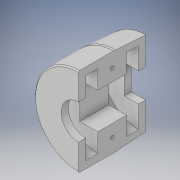
# Autodesk Inventor part: cameraHolder
Saved by Autodesk Inventor 2019.3 (Build 233278000, 278)
## iProperties
Created: 2019-10-29
Part Number: cameraHolder
Material: Generic
Document SubType Name: Modeling
Designer: Ayaz
Density: 1 g/cm^3
Appearance: Default
Author: Ayaz
Autodesk Inventor part; units mm, degrees
ref_plane "YZ Plane" through (0, 0, 0) normal (1, 0, 0) x (0, 1, 0)
ref_plane "XZ Plane" through (0, 0, 0) normal (0, 1, 0) x (-1, 0, 0)
ref_plane "XY Plane" through (0, 0, 0) normal (0, 0, 1) x (1, 0, 0)
sketch "Sketch1" plane through (0, 0, 0) normal (0, 1, 0) x (-1, 0, 0)
  line L0 (0, 0) -> (0, 36.83)
  line L1 (0, 0) -> (-56, 0)
  line L2 (-56, 0) -> (-56, 34.9885)
  line L3 (11.2, 0) -> (-67.2, 0) projected
  line L4 (-50, 30.1718) -> (-50, 6)
  line L5 (-6, 6) -> (-6, 30.7506)
  line L6 (-6, 30.7506) -> (-50, 30.1718)
  line L7 (-28, 0) -> (-28, 30.4612)
  line L8 (-16, 0) -> (-16, 30.619)
  line L9 (-40, 0) -> (-40, 30.3033)
  line L10 (-50, 6) -> (-40, 6)
  line L11 (-16, 6) -> (-6, 6)
  line L12 (0, 36.83) -> (-30, 36.83)
  line L13 (-30, 36.83) -> (-56, 34.9885)
  dimension "d1" = 34.9885
  dimension "d8" = 36.83
  dimension "d10" = 56
  dimension "d22" = 28
  dimension "d23" = 12
  dimension "d24" = 12
  dimension "d29" = 30
  constraints: 26 end point, 4 point on line, 2 midpoint, 2 parallel, 2 vertical, 1 horizontal, 1 perpendicular
  measures "d1" distance of L1.end L2.end
  measures "d8" distance of L0.start L0.end
  measures "d10" distance of L0.start L1.end
  measures "d22" distance between parallel lines of L0 L7
  measures "d23" distance between parallel lines of L7 L8
  measures "d24" distance between parallel lines of L7 L9
  measures "d29" distance of L0.end L12.end
revolve "Revolution1" add sketch "Sketch1" angle 180 about axis through (-10, 0, 0) along (-1, 0, 0) contours L1 L8 L11 L5 L6 L4 L10 L9 L2 L13 L12 L0 | L1 L7 L6 L8 | L1 L9 L6 L7
ref_plane "Work Plane1" through (6, 0, 0) normal (-1, 0, 0) x (0, 0, -1)
sketch "Sketch3" plane through (6, 0, 0) normal (-1, 0, 0) x (0, 0, -1)
  line L0 (-15, 15) -> (15, 15)
  line L1 (15, 15) -> (15, -15)
  line L2 (15, -15) -> (-15, -15)
  line L3 (-15, -15) -> (-15, 15)
  line L4 (-15, 15) -> (15, -15) construction
  line L5 (15, 15) -> (-15, -15) construction
  point P0 (0, 0)
  dimension "d12" = 30
  dimension "d13" = 30
  constraints: 12 end point, 2 midpoint, 2 parallel, 1 horizontal, 1 perpendicular
  measures "d12" distance of L1.end L2.end
  measures "d13" distance of L0.end L1.end
extrude "Extrusion2" cut sketch "Sketch3" against normal blind 44
sketch "Sketch4" plane through (0, 0, 0) normal (-1, 0, 0) x (0, 0, -1)
  circle A0 centre (0, 0) radius 14.5
  point P0 (0, 0)
  dimension "d16" = 29
  constraints: 1 centre point, 1 coincident
  measures "d16" diameter of A0
extrude "Extrusion3" cut sketch "Sketch4" against normal blind 6
sketch "Sketch5" plane through (56, 0, 0) normal (1, 0, 0) x (0, 0, -1)
  line L0 (12, -12) -> (-12, -12)
  line L1 (-12, -12) -> (-12, 12)
  line L2 (-12, 12) -> (12, 12)
  line L3 (12, 12) -> (12, -12)
  line L4 (12, -12) -> (-12, 12) construction
  line L5 (-12, -12) -> (12, 12) construction
  point P0 (0, 0)
  dimension "d25" = 24
  dimension "d26" = 24
  constraints: 12 end point, 2 midpoint, 2 parallel, 1 horizontal, 1 perpendicular
  measures "d25" distance of L1.end L2.end
  measures "d26" distance of L0.end L1.end
extrude "Extrusion4" cut sketch "Sketch5" against normal blind 6
chamfer "Chamfer2" distance 1 angle 45 1 edges at (30, 36.83, 0)
chamfer "Chamfer3" distance 1 angle 45 1 edges at (0, 36.83, 0)
sketch "Sketch6" plane through (16, 0, 15) normal (0, -1, 0) x (1, 0, 0)
  line L0 (-16, 20.83) -> (-15, 21.83) projected
  line L1 (-16, -0.5) -> (-16, 20.83) projected
  line L2 (-16, -0.5) -> (-10, -0.5) projected
  line L3 (-10, -0.5) -> (-10, 15.7506) projected
  line L4 (-10, 15.7506) -> (0, 15.619) projected
  line L5 (0, 15.619) -> (0, 0) projected
  line L6 (0, 0) -> (24, 0) projected
  line L7 (24, 0) -> (24, 15.3033) projected
  line L8 (24, 15.3033) -> (34, 15.1718) projected
  line L9 (34, 15.1718) -> (34, -3) projected
  line L10 (34, -3) -> (40, -3) projected
  line L11 (40, 19.9885) -> (40, -3) projected
  line L12 (14.9975, 21.7594) -> (40, 19.9885) projected
  line L13 (13, 21.83) -> (14.9975, 21.7594) projected
  line L14 (-15, 21.83) -> (13, 21.83) projected
  line L15 (-16, -15) -> (40, -15)
  line L16 (40, -3) -> (40, -27) projected
  line L17 (13, -15) -> (38, -15) construction
  line L18 (12, -15) -> (12, 10)
  line L19 (13, -51.83) -> (13, 21.83) projected
  line L20 (12, -15) -> (37, -15) construction
  circle A0 centre (12, 10) radius 1.5
  dimension "d46" = 25
  dimension "d47" = 90
  dimension "d48" = 3
  constraints: 8 end point, 2 horizontal, 2 midpoint, 1 centre point, 1 coincident, 1 parallel, 1 perpendicular
  measures "d46" distance of L18.start L18.end
  measures "d47" angle of L20 L18
  measures "d48" diameter of A0
extrude "Extrusion5" cut sketch "Sketch6" against normal blind 3 contours A0 L19 | L19 A0
mirror "Mirror1" about plane through (0, 0, 0) normal (0, 0, 1) of "Extrusion5"
equation "\"d8\" = 0.5 * pipeID"
equation "\"d22\" = 0.5 * d10"
equation "\"d23\" = 2 * wallTh"
equation "\"d24\" = 2 * wallTh"
equation "\"d29\" = 5 * wallTh"
equation "\"d17\" = wallTh"
equation "\"d27\" = wallTh"
equation "\"pipeID\" = 73.66"
equation "\"wallTh\" = 6"
equation "\"taper\" = 0.95"
equation "\"d11\" = -wallTh"
body "Solid1"
